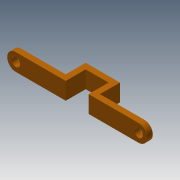
# Autodesk Inventor part: tahlo7
Saved by Autodesk Inventor 2013 (Build 170138000, 138)
## iProperties
Created: 2013-03-24
Part Number: tahlo7
Material: Generic
Document SubType Name: Modeling
Designer: idle-rug
Density: 1 g/cm^3
Author: idle-rug
Autodesk Inventor part; units mm, degrees
ref_plane "YZ Plane" through (0, 0, 0) normal (1, 0, 0) x (0, 1, 0)
ref_plane "XZ Plane" through (0, 0, 0) normal (0, 1, 0) x (-1, 0, 0)
ref_plane "XY Plane" through (0, 0, 0) normal (0, 0, 1) x (1, 0, 0)
sketch "Sketch2" plane through (0, 0, 0) normal (0, 1, 0) x (-1, 0, 0)
  line L0 (21.5, 3) -> (-21.5, 3)
  line L1 (-21.5, 3) -> (-21.5, -3)
  line L2 (-21.5, -3) -> (21.5, -3)
  line L3 (21.5, -3) -> (21.5, 3)
  line L4 (21.5, 3) -> (-21.5, -3) construction
  line L5 (-21.5, 3) -> (21.5, -3) construction
  circle A0 centre (-21.5, 0) radius 3
  circle A1 centre (21.5, 0) radius 3
  point P0 (0, 0)
  dimension "d6" = 43
  dimension "d7" = 6
  constraints: 12 end point, 4 midpoint, 2 parallel, 2 vertical alignment, 1 horizontal, 1 perpendicular, 4 other
  measures "d6" distance of L2.end L1.end
  measures "d7" distance of L1.end L0.end
extrude "Extrusion1" add sketch "Sketch2" along normal blind 2
sketch "Sketch3" plane through (0, 2, 0) normal (0, 1, 0) x (1, 0, 0)
  line L0 (-21.5, -3) -> (21.5, -3) projected
  line L1 (5, 3) -> (-5, 3)
  line L2 (-5, 3) -> (-5, -3)
  line L3 (-5, -3) -> (5, -3)
  line L4 (5, -3) -> (5, 3)
  line L5 (5, 3) -> (-5, -3) construction
  line L6 (-5, 3) -> (5, -3) construction
  point P0 (0, 0)
  dimension "d10" = 10
  constraints: 12 end point, 2 midpoint, 2 parallel, 1 horizontal, 1 perpendicular, 1 point on line
  measures "d10" distance of L3.end L2.end
extrude "Extrusion2" add sketch "Sketch3" along normal blind 7
sketch "Sketch4" plane through (0, 0, 0) normal (0, -1, 0) x (1, 0, 0)
  line L0 (-21.5, 3) -> (21.5, 3) projected
  line L1 (4, -3) -> (-4, -3)
  line L2 (-4, -3) -> (-4, 3)
  line L3 (-4, 3) -> (4, 3)
  line L4 (4, 3) -> (4, -3)
  line L5 (4, -3) -> (-4, 3) construction
  line L6 (-4, -3) -> (4, 3) construction
  point P0 (0, 0)
  dimension "d13" = 8
  constraints: 12 end point, 2 midpoint, 2 parallel, 1 horizontal, 1 perpendicular, 1 point on line
  measures "d13" distance of L2.end L3.end
extrude "Extrusion3" cut sketch "Sketch4" against normal blind 7
sketch "Sketch5" plane through (5, 2, 3) normal (1, 0, 0) x (0, 0, -1)
  line L0 (6, 0) -> (0, 0) projected
  line L1 (6, 0) -> (6, 7) projected
  line L2 (0, 7) -> (6, 7) projected
  line L3 (0, 0) -> (0, 7) projected
  point P0 (3, -2)
extrude "Extrusion4" add sketch "Sketch5" along normal blind 1
sketch "Sketch6" plane through (-5, 2, -3) normal (-1, 0, 0) x (0, 0, 1)
  line L0 (6, 0) -> (0, 0) projected
  line L1 (6, 0) -> (6, 7) projected
  line L2 (0, 7) -> (6, 7) projected
  line L3 (0, 0) -> (0, 7) projected
  point P0 (3, -2)
extrude "Extrusion5" add sketch "Sketch6" along normal blind 1
sketch "Sketch7" plane through (0, 2, 0) normal (0, 1, 0) x (1, 0, 0)
  arc A0 (21.5, -3) -> (21.5, 3) centre (21.5, 0) ccw projected
  circle A1 centre (21.5, 0) radius 1.5
  point P0 (0, 0)
  dimension "d20" = 3
  constraints: 1 centre point, 1 coincident
  measures "d20" diameter of A1
sketch "Sketch8" plane through (0, 2, 0) normal (0, 1, 0) x (1, 0, 0)
  arc A0 (-21.5, 3) -> (-21.5, -3) centre (-21.5, 0) ccw projected
  circle A1 centre (-21.5, 0) radius 1.5
  point P0 (0, 0)
  dimension "d21" = 3
  constraints: 1 centre point, 1 coincident
  measures "d21" diameter of A1
extrude "Extrusion6" cut sketch "Sketch8" against normal blind 2
extrude "Extrusion7" cut sketch "Sketch7" against normal blind 2
body "Solid1"
